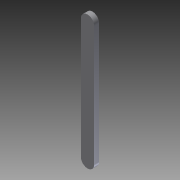
# Autodesk Inventor part: top bottom link
Saved by Autodesk Inventor 2012 (Build 160160000, 160)
## iProperties
Created: 2012-01-14
Part Number: top bottom link
Material: Default
Document SubType Name: Modeling
Designer: Antonella Wilby
Density: 1 g/cm^3
Author: Antonella Wilby
Autodesk Inventor part; units mm, degrees
ref_plane "YZ Plane" through (0, 0, 0) normal (1, 0, 0) x (0, 1, 0)
ref_plane "XZ Plane" through (0, 0, 0) normal (0, 1, 0) x (-1, 0, 0)
ref_plane "XY Plane" through (0, 0, 0) normal (0, 0, 1) x (1, 0, 0)
sketch "Sketch1" plane through (0, 0, 0) normal (0, 0, 1) x (1, 0, 0)
  line L0 (-8.89, 0) -> (8.89, 0) projected
  line L1 (0, -88.9) -> (0, 88.9) projected
  line L2 (-6.35, 57.15) -> (6.35, 57.15) construction
  line L3 (6.35, 57.15) -> (6.35, -57.15)
  line L4 (6.35, -57.15) -> (-6.35, -57.15) construction
  line L5 (-6.35, -57.15) -> (-6.35, 57.15)
  arc A0 (6.35, 57.15) -> (-6.35, 57.15) centre (0, 57.15) ccw
  arc A1 (-6.35, -57.15) -> (6.35, -57.15) centre (0, -57.15) ccw
  point P0 (0, 0)
  point P1 (-6.35, 0)
  dimension "d0" = 12.7
  dimension "d1" = 114.3
  constraints: 8 end point, 4 point on circle, 3 midpoint, 2 centre point, 2 parallel, 1 coincident, 1 horizontal, 1 horizontal alignment, 1 perpendicular, 1 vertical alignment
  measures "d0" distance between parallel lines of L3 L5
  measures "d1" distance of L4.end L2.start
extrude "Extrusion1" add sketch "Sketch1" along normal mid plane 4.7625
body "Solid1"
